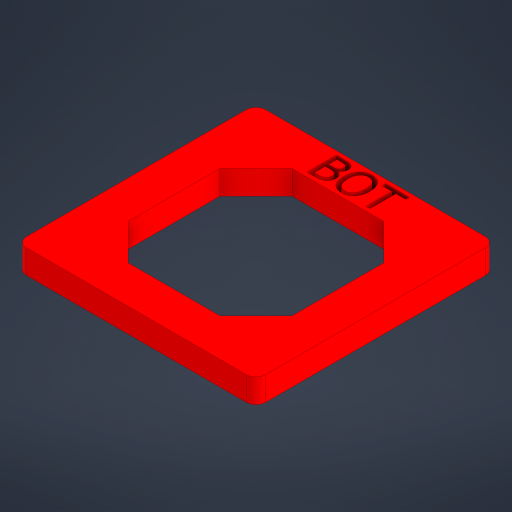
# Autodesk Inventor part: Cube 1x1 V5 Bot Press
Saved by Autodesk Inventor 2023.4 (Build 274418000, 418)
## iProperties
Created: 2022-07-25
Part Number: Cube 1x1 V5 Bot Press
Material: Generic
Document SubType Name: Modeling
Designer: xSibe
Density: 1 g/cm^3
Appearance: Plastic Red
Author: xSibe
Autodesk Inventor part; units mm, degrees
ref_plane "YZ Plane" through (0, 0, 0) normal (1, 0, 0) x (0, 1, 0)
ref_plane "XZ Plane" through (0, 0, 0) normal (0, 1, 0) x (-1, 0, 0)
ref_plane "XY Plane" through (0, 0, 0) normal (0, 0, 1) x (1, 0, 0)
sketch "Sketch1" plane through (0, 0, 0) normal (0, 1, 0) x (-1, 0, 0)
  line L0 (24.9, 24.9) -> (-24.9, 24.9)
  line L1 (-24.9, 24.9) -> (-24.9, -24.9)
  line L2 (-24.9, -24.9) -> (24.9, -24.9)
  line L3 (24.9, -24.9) -> (24.9, 24.9)
  line L4 (24.9, 24.9) -> (-24.9, -24.9) construction
  line L5 (-24.9, 24.9) -> (24.9, -24.9) construction
  line L6 (17.05, 17.05) -> (-17.05, 17.05)
  line L7 (-17.05, 17.05) -> (-17.05, -17.05)
  line L8 (-17.05, -17.05) -> (17.05, -17.05)
  line L9 (17.05, -17.05) -> (17.05, 17.05)
  line L10 (24.9, -24.9) -> (21.9, -24.9)
  line L11 (21.9, -24.9) -> (21.9, -21.9)
  line L12 (21.9, -21.9) -> (24.9, -21.9)
  line L13 (24.9, -21.9) -> (24.9, -24.9)
  circle A0 centre (21.9, -21.9) radius 1.875
  circle A1 centre (21.9, -21.9) radius 2.1063
  circle A2 centre (21.9, -21.9) radius 2.7813
  line L14 (24.9, -24.9) -> (14.4, -24.9)
  line L15 (14.4, -24.9) -> (14.4, -14.4)
  line L16 (14.4, -14.4) -> (24.9, -14.4)
  line L17 (24.9, -14.4) -> (24.9, -24.9)
  line L18 (24.9, -14.4) -> (20.8, -14.4)
  circle A3 centre (20.8, -14.4) radius 2.0725
  circle A4 centre (14.4, -20.8) radius 2.0725
  line L19 (24.9, -24.9) -> (17.05, -24.9)
  line L20 (17.05, -24.9) -> (17.05, -22.55)
  line L21 (22.55, -17.05) -> (24.9, -17.05)
  line L22 (24.9, -17.05) -> (24.9, -24.9)
  line L23 (22.55, -17.05) -> (17.05, -22.55)
  circle A5 centre (21.9, 21.9) radius 2.7813
  circle A6 centre (21.9, 21.9) radius 2.1063
  circle A7 centre (21.9, 21.9) radius 1.875
  circle A8 centre (14.4, 20.8) radius 2.0725
  circle A9 centre (20.8, 14.4) radius 2.0725
  line L24 (17.05, 22.55) -> (22.55, 17.05)
  line L25 (24.9, 17.05) -> (22.55, 17.05)
  line L26 (17.05, 22.55) -> (17.05, 24.9)
  circle A10 centre (-21.9, 21.9) radius 2.7813
  circle A11 centre (-21.9, 21.9) radius 2.1063
  circle A12 centre (-21.9, 21.9) radius 1.875
  circle A13 centre (-20.8, 14.4) radius 2.0725
  circle A14 centre (-14.4, 20.8) radius 2.0725
  line L27 (-22.55, 17.05) -> (-17.05, 22.55)
  line L28 (-17.05, 24.9) -> (-17.05, 22.55)
  line L29 (-22.55, 17.05) -> (-24.9, 17.05)
  circle A15 centre (-21.9, -21.9) radius 2.7813
  circle A16 centre (-21.9, -21.9) radius 2.1063
  circle A17 centre (-21.9, -21.9) radius 1.875
  circle A18 centre (-14.4, -20.8) radius 2.0725
  circle A19 centre (-20.8, -14.4) radius 2.0725
  line L30 (-17.05, -22.55) -> (-22.55, -17.05)
  line L31 (-24.9, -17.05) -> (-22.55, -17.05)
  line L32 (-17.05, -22.55) -> (-17.05, -24.9)
  line L33 (17.05, -22.55) -> (-17.05, -22.55)
  line L34 (-22.55, -17.05) -> (-22.55, 17.05)
  line L35 (-17.05, 22.55) -> (17.05, 22.55)
  line L36 (22.55, 17.05) -> (22.55, -17.05)
  point P0 (0, 0)
  point P1 (-15.5103, -22.55)
  point P2 (14.4, -22.8725)
  point P3 (13.2897, -22.55)
  point P4 (-13.2897, -22.55)
  point P5 (-22.55, -15.5103)
  point P6 (-22.55, -13.2897)
  point P7 (-22.55, 13.2897)
  point P8 (-22.55, 15.5103)
  point P9 (-15.5103, 22.55)
  point P10 (-13.2897, 22.55)
  point P11 (13.2897, 22.55)
  point P12 (15.5103, 22.55)
  point P13 (22.55, -15.5103)
  point P14 (22.55, 15.5103)
  point P15 (22.55, 13.2897)
  point P16 (22.55, -13.2897)
  point P17 (15.5103, -22.55)
  dimension "d0" = 49.8
  dimension "d1" = 49.8
  dimension "d2" = 7.85
  dimension "d3" = 3
  dimension "d4" = 3
  dimension "d5" = 3.75
  dimension "d6" = 4.2125
  dimension "d7" = 0.675
  dimension "d8" = 10.5
  dimension "d9" = 10.5
  dimension "d10" = 4.1
  dimension "d11" = 4.145
  dimension "d12" = 7.85
  dimension "d13" = 7.85
  dimension "d14" = 5.5
  dimension "d15" = 5.5
  dimension "d18" = 360
  constraints: 74 end point, 20 centre point, 10 parallel, 7 perpendicular, 6 coincident, 4 horizontal, 3 point on line, 2 midpoint, 1 symmetric about line, 69 other
  measures "d0" distance of L2.end L1.end
  measures "d1" distance of L1.end L0.end
  measures "d2" distance between parallel lines of L3 L9
  measures "d3" distance of L11.end L12.end
  measures "d4" distance of L10.end L11.end
  measures "d5" diameter of A0
  measures "d6" diameter of A1
  measures "d7" radial gap between concentric circles of A1 A2
  measures "d8" distance of L15.end L16.end
  measures "d9" distance of L14.end L15.end
  measures "d10" distance of L16.end L18.end
  measures "d11" diameter of A3
  measures "d12" distance of point (17.05, -17.05) L21.end
  measures "d13" distance of L19.end point (17.05, -17.05)
  measures "d14" distance of L21.start point (17.05, -17.05)
  measures "d15" distance of L20.end point (17.05, -17.05)
extrude "Extrusion1" add sketch "Sketch1" along normal blind 7.7 contours L3 L25 L24 L26 L0 | L26 L35 A8 A14 L28 L0 | L3 L16 A3 L36 A9 L25 | L28 L27 L29 L1 L0 | L3 L21 L36 A3 L16 | L3 L12 A2 L11 L2 L20 L23 L21 | L29 L34 A13 A19 L31 L1 | L3 L2 L11 A2 L12 | L31 L30 L32 L2 L1 | A2 L11 A1 L12 | L12 A1 L11 A2 | L20 L2 L15 A4 L33 | A1 L11 A0 L12 | L12 A0 L11 A1 | L32 L33 A18 A4 L15 L2 | A0 L11 L12 | L12 L11 A0 | A5 | A6 | A7 | A10 | A11 | A12 | A15 | A16 | A17
extrude "Extrusion2" add sketch "Sketch1" against normal up to surface (7.7 mm away) from surface at 7.7 contours L26 L35 A8 A14 L28 L0 | L3 L16 A3 L36 A9 L25 | L24 L36 A9 A3 L16 L9 L6 L7 L8 L15 A4 L33 A18 L30 L34 A19 A13 L27 L35 A14 A8 | L3 L21 L36 A3 L16 | A3 L36 L16 | L16 L36 A3 | L36 A9 | A9 L36 | L29 L34 A13 A19 L31 L1 | L23 L33 A4 L15 L8 L9 L16 A3 L36 | L36 A3 L16 | L16 A3 L36 | L34 A13 | A13 L34 | L20 L2 L15 A4 L33 | L32 L33 A18 A4 L15 L2 | L34 A19 | A19 L34
chamfer "Chamfer1" [suppressed]
fillet "Fillet1" radius 2 4 edges at (24.9, 3.85, 24.9) (24.9, 3.85, -24.9) (-24.9, 3.85, -24.9) (-24.9, 3.85, 24.9)
chamfer "Chamfer2" distance 0.025 angle 45 8 edges at (0, 7.7, 24.9) (24.3142, 7.7, 24.3142) (24.9, 7.7, 0) (24.3142, 7.7, -24.3142) (0, 7.7, -24.9) (-24.3142, 7.7, -24.3142) (-24.9, 7.7, 0) (-24.3142, 7.7, 24.3142)
extrude "Extrusion3" cut sketch "Sketch1" along normal blind 3 contours A1 L11 A0 L12 | L12 A0 L11 A1 | A0 L11 L12 | L12 L11 A0 | A6 | A7 | A11 | A12 | A16 | A17
extrude "Extrusion4" cut sketch "Sketch1" along normal up to surface (4.7 mm away) from surface at 3 contours A0 L11 L12 | L12 L11 A0 | A7 | A12 | A17
sketch "Sketch2" plane through (0, 7.7, 24.9) normal (0, 0, 1) x (1, 0, 0)
  line L0 (-8.2534, -7.5059) -> (8.2534, -7.5059) construction
  line L1 (8.2534, -7.5059) -> (8.2534, -0.2191) construction
  line L2 (8.2534, -0.2191) -> (-8.2534, -0.2191) construction
  line L3 (-8.2534, -0.2191) -> (-8.2534, -7.5059) construction
  line L4 (-22.9, -3.8625) -> (22.9, -3.8625)
  line L5 (-8.2534, -3.8625) -> (8.2534, -3.8625)
  line L6 (-22.9, -0.025) -> (22.9, -0.025) projected
  line L7 (-22.9, -7.7) -> (-22.9, -0.025) projected
  line L8 (-22.9, -7.7) -> (22.9, -7.7) projected
  line L9 (22.9, -0.025) -> (22.9, -7.7) projected
  point P0 (0, -7.7)
  point P1 (0, -3.8625)
  constraints: 6 midpoint, 4 end point, 1 horizontal, 2 other
extrude "Extrusion5" [suppressed]
pattern_circular "Circular Pattern1" [suppressed]
sketch "Sketch3" plane through (0, 7.7, 0) normal (0, 1, 0) x (1, 0, 0)
  circle A0 centre (21.9, 21.9) radius 1.875 projected
  circle A1 centre (-21.9, -21.9) radius 1.875 projected
  circle A2 centre (-21.9, 21.9) radius 1.875 projected
  circle A3 centre (21.9, -21.9) radius 1.875 projected
  circle A4 centre (-14.4, -20.8) radius 2.0725 projected
  circle A5 centre (14.4, 20.8) radius 2.0725 projected
  circle A6 centre (-14.4, 20.8) radius 2.0725 projected
  line L0 (17.05, -17.05) -> (17.05, 17.05) projected
  line L1 (-17.05, -17.05) -> (17.05, -17.05) projected
  line L2 (-17.05, 17.05) -> (-17.05, -17.05) projected
  line L3 (17.05, 17.05) -> (-17.05, 17.05) projected
  circle A7 centre (14.4, -20.8) radius 2.0725 projected
  line L4 (22.9, -24.875) -> (-22.9, -24.875) projected
  arc A8 (22.9, -24.875) -> (24.875, -22.9) centre (22.9, -22.9) ccw projected
  line L5 (24.875, 22.9) -> (24.875, -22.9) projected
  arc A9 (24.875, 22.9) -> (22.9, 24.875) centre (22.9, 22.9) ccw projected
  line L6 (-22.9, 24.875) -> (22.9, 24.875) projected
  arc A10 (-22.9, 24.875) -> (-24.875, 22.9) centre (-22.9, 22.9) ccw projected
  line L7 (-24.875, -22.9) -> (-24.875, 22.9) projected
  arc A11 (-24.875, -22.9) -> (-22.9, -24.875) centre (-22.9, -22.9) ccw projected
  point P0 (0, 0)
extrude "Extrusion6" add sketch "Sketch3" against normal up to surface (7.7 mm away) contours A0 | A1 | A2 | A3 | L4 A11 L7 A10 L6 A9 L5 A8
sketch "Sketch4" plane through (0, 7.7, 0) normal (0, 1, 0) x (1, 0, 0)
  circle A0 centre (14.4, 20.8) radius 2.0725 projected
  circle A1 centre (-14.4, 20.8) radius 2.0725 projected
  circle A2 centre (-14.4, -20.8) radius 2.0725 projected
  circle A3 centre (14.4, -20.8) radius 2.0725 projected
  line L0 (22.9, -24.875) -> (-22.9, -24.875) projected
  arc A4 (22.9, -24.875) -> (24.875, -22.9) centre (22.9, -22.9) ccw projected
  line L1 (24.875, 22.9) -> (24.875, -22.9) projected
  arc A5 (24.875, 22.9) -> (22.9, 24.875) centre (22.9, 22.9) ccw projected
  line L2 (-22.9, 24.875) -> (22.9, 24.875) projected
  arc A6 (-22.9, 24.875) -> (-24.875, 22.9) centre (-22.9, 22.9) ccw projected
  line L3 (-24.875, -22.9) -> (-24.875, 22.9) projected
  arc A7 (-24.875, -22.9) -> (-22.9, -24.875) centre (-22.9, -22.9) ccw projected
  point P0 (0, 0)
extrude "Extrusion7" add sketch "Sketch4" against normal blind 5.7 contours A0 | A1 | A2 | A3
chamfer "Chamfer3" distance 7.5 angle 45 4 edges at (-17.05, 3.85, 17.05) (17.05, 3.85, 17.05) (17.05, 3.85, -17.05) (-17.05, 3.85, -17.05)
sketch "Sketch5" plane through (0, 7.7, 0) normal (0, 1, 0) x (1, 0, 0)
  line L0 (-9.55, -17.05) -> (9.55, -17.05) projected
  line L1 (-17.05, -9.55) -> (-9.55, -17.05) projected
  line L2 (-17.05, 9.55) -> (-17.05, -9.55) projected
  line L3 (-9.55, 17.05) -> (-17.05, 9.55) projected
  line L4 (9.55, 17.05) -> (-9.55, 17.05) projected
  line L5 (17.05, 9.55) -> (9.55, 17.05) projected
  line L6 (17.05, -9.55) -> (17.05, 9.55) projected
  line L7 (9.55, -17.05) -> (17.05, -9.55) projected
  line L8 (22.9, -24.875) -> (-22.9, -24.875) projected
  arc A0 (22.9, -24.875) -> (24.875, -22.9) centre (22.9, -22.9) ccw projected
  line L9 (24.875, 22.9) -> (24.875, -22.9) projected
  arc A1 (24.875, 22.9) -> (22.9, 24.875) centre (22.9, 22.9) ccw projected
  line L10 (-22.9, 24.875) -> (22.9, 24.875) projected
  arc A2 (-22.9, 24.875) -> (-24.875, 22.9) centre (-22.9, 22.9) ccw projected
  line L11 (-24.875, -22.9) -> (-24.875, 22.9) projected
  arc A3 (-24.875, -22.9) -> (-22.9, -24.875) centre (-22.9, -22.9) ccw projected
  line L12 (22.9, 24.9) -> (-22.9, 24.9) projected
  arc A4 (-22.9, 24.875) -> (-24.875, 22.9) centre (-22.9, 22.9) ccw projected
  arc A5 (-22.9, 24.9) -> (-24.9, 22.9) centre (-22.9, 22.9) ccw projected
  line L13 (-24.9, 22.9) -> (-24.9, -22.9) projected
  arc A6 (-24.9, -22.9) -> (-22.9, -24.9) centre (-22.9, -22.9) ccw projected
  arc A7 (-24.9, -22.9) -> (-22.9, -24.9) centre (-22.9, -22.9) ccw projected
  line L14 (-22.9, -24.9) -> (22.9, -24.9) projected
  line L15 (-22.9, -24.9) -> (22.9, -24.9) projected
  arc A8 (22.9, -24.9) -> (24.9, -22.9) centre (22.9, -22.9) ccw projected
  arc A9 (22.9, -24.9) -> (24.9, -22.9) centre (22.9, -22.9) ccw projected
  line L16 (24.9, -22.9) -> (24.9, 22.9) projected
  line L17 (24.9, -22.9) -> (24.9, 22.9) projected
  arc A10 (24.9, 22.9) -> (22.9, 24.9) centre (22.9, 22.9) ccw projected
  arc A11 (24.9, 22.9) -> (22.9, 24.9) centre (22.9, 22.9) ccw projected
  line L18 (0, 17.05) -> (0, 24.9)
  line L19 (-10, 17.05) -> (10, 17.05)
  line L20 (10, 17.05) -> (10, 24.9)
  line L21 (10, 24.9) -> (-10, 24.9)
  line L22 (-10, 24.9) -> (-10, 17.05)
  line L23 (-10, 17.05) -> (10, 24.9) construction
  line L24 (10, 17.05) -> (-10, 24.9) construction
  line L25 (-10, 24.9) -> (10, 24.9) construction
  line L26 (10, 24.9) -> (10, 17.05) construction
  line L27 (10, 17.05) -> (-10, 17.05) construction
  line L28 (-10, 17.05) -> (-10, 24.9) construction
  spline S0 degree 2 poles (-3.1365, 19.7985) (-3.1365, 19.3437) (-3.4825, 18.6467) (-3.7692, 18.4193) knots 0 0 0 1 2 2 2
  spline S1 degree 2 poles (-3.7692, 18.4193) (-4.1153, 18.1524) (-4.9013, 17.925) (-5.5241, 17.925) knots 0 0 0 1 2 2 2
  line L29 (-5.5241, 17.925) -> (-7.274, 17.925)
  line L30 (-7.274, 17.925) -> (-7.274, 24.025)
  line L31 (-7.274, 24.025) -> (-5.6576, 24.025)
  spline S2 degree 2 poles (-5.6576, 24.025) (-5.0051, 24.025) (-4.3526, 23.941) (-4.056, 23.7778) knots 0 0 0 1 2 2 2
  spline S3 degree 2 poles (-4.056, 23.7778) (-3.7248, 23.6048) (-3.4232, 23.0363) (-3.4232, 22.6508) knots 0 0 0 1 2 2 2
  spline S4 degree 2 poles (-3.4232, 22.6508) (-3.4232, 22.2207) (-3.878, 21.5385) (-4.2784, 21.3457) knots 0 0 0 1 2 2 2
  line L32 (-4.2784, 21.3457) -> (-4.2784, 21.3161)
  spline S5 degree 2 poles (-4.2784, 21.3161) (-3.7346, 21.1678) (-3.1365, 20.3818) (-3.1365, 19.7985) knots 0 0 0 1 2 2 2
  spline S6 degree 2 poles (-3.9818, 19.7639) (-3.9818, 20.1099) (-4.1795, 20.5548) (-4.4761, 20.713) knots 0 0 0 1 2 2 2
  spline S7 degree 2 poles (-4.4761, 20.713) (-4.6689, 20.8119) (-5.1237, 20.8712) (-5.5439, 20.8712) knots 0 0 0 1 2 2 2
  line L33 (-5.5439, 20.8712) -> (-6.4633, 20.8712)
  line L34 (-6.4633, 20.8712) -> (-6.4633, 18.6171)
  line L35 (-6.4633, 18.6171) -> (-5.8059, 18.6171)
  spline S8 degree 2 poles (-5.8059, 18.6171) (-5.272, 18.6171) (-4.659, 18.7159) (-4.4218, 18.8741) knots 0 0 0 1 2 2 2
  spline S9 degree 2 poles (-4.4218, 18.8741) (-4.1944, 19.0372) (-3.9818, 19.4426) (-3.9818, 19.7639) knots 0 0 0 1 2 2 2
  spline S10 degree 2 poles (-4.2685, 22.5371) (-4.2685, 22.7546) (-4.4168, 23.0808) (-4.5799, 23.1748) knots 0 0 0 1 2 2 2
  spline S11 degree 2 poles (-4.5799, 23.1748) (-4.7777, 23.2835) (-5.2572, 23.3329) (-5.6872, 23.3329) knots 0 0 0 1 2 2 2
  line L36 (-5.6872, 23.3329) -> (-6.4633, 23.3329)
  line L37 (-6.4633, 23.3329) -> (-6.4633, 21.5484)
  line L38 (-6.4633, 21.5484) -> (-5.5439, 21.5484)
  spline S12 degree 2 poles (-5.5439, 21.5484) (-5.1632, 21.5484) (-4.8024, 21.6275) (-4.6096, 21.7511) knots 0 0 0 1 2 2 2
  spline S13 degree 2 poles (-4.6096, 21.7511) (-4.4218, 21.8697) (-4.2685, 22.2504) (-4.2685, 22.5371) knots 0 0 0 1 2 2 2
  spline S14 degree 2 poles (1.9847, 23.328) (2.3308, 22.9227) (2.7163, 21.7363) (2.7163, 20.975) knots 0 0 0 1 2 2 2
  spline S15 degree 2 poles (2.7163, 20.975) (2.7163, 20.2335) (2.3406, 19.0323) (1.9847, 18.6269) knots 0 0 0 1 2 2 2
  spline S16 degree 2 poles (1.9847, 18.6269) (1.609, 18.2018) (0.6154, 17.7965) (0.0173, 17.7965) knots 0 0 0 1 2 2 2
  spline S17 degree 2 poles (0.0173, 17.7965) (-0.6006, 17.7965) (-1.5893, 18.2167) (-1.9501, 18.6269) knots 0 0 0 1 2 2 2
  spline S18 degree 2 poles (-1.9501, 18.6269) (-2.3011, 19.0323) (-2.6768, 20.2236) (-2.6768, 20.975) knots 0 0 0 1 2 2 2
  spline S19 degree 2 poles (-2.6768, 20.975) (-2.6768, 21.7412) (-2.2962, 22.9078) (-1.9452, 23.328) knots 0 0 0 1 2 2 2
  spline S20 degree 2 poles (-1.9452, 23.328) (-1.5893, 23.7333) (-0.5957, 24.1535) (0.0173, 24.1535) knots 0 0 0 1 2 2 2
  spline S21 degree 2 poles (0.0173, 24.1535) (0.6402, 24.1535) (1.6387, 23.7185) (1.9847, 23.328) knots 0 0 0 1 2 2 2
  spline S22 degree 2 poles (1.871, 20.975) (1.871, 21.5781) (1.609, 22.5124) (1.3718, 22.8188) knots 0 0 0 1 2 2 2
  spline S23 degree 2 poles (1.3718, 22.8188) (1.1295, 23.1352) (0.4474, 23.4516) (0.0222, 23.4516) knots 0 0 0 1 2 2 2
  spline S24 degree 2 poles (0.0222, 23.4516) (-0.4177, 23.4516) (-1.0801, 23.1451) (-1.3322, 22.8188) knots 0 0 0 1 2 2 2
  spline S25 degree 2 poles (-1.3322, 22.8188) (-1.5744, 22.5074) (-1.8315, 21.5682) (-1.8315, 20.975) knots 0 0 0 1 2 2 2
  spline S26 degree 2 poles (-1.8315, 20.975) (-1.8315, 19.7738) (-0.8231, 18.4984) (0.0222, 18.4984) knots 0 0 0 1 2 2 2
  spline S27 degree 2 poles (0.0222, 18.4984) (0.8675, 18.4984) (1.871, 19.7738) (1.871, 20.975) knots 0 0 0 1 2 2 2
  line L39 (5.0298, 17.925) -> (5.0298, 23.3033)
  line L40 (5.0298, 23.3033) -> (2.9833, 23.3033)
  line L41 (2.9833, 23.3033) -> (2.9833, 24.025)
  line L42 (2.9833, 24.025) -> (7.887, 24.025)
  line L43 (7.887, 24.025) -> (7.887, 23.3033)
  line L44 (7.887, 23.3033) -> (5.8405, 23.3033)
  line L45 (5.8405, 23.3033) -> (5.8405, 17.925)
  line L46 (5.8405, 17.925) -> (5.0298, 17.925)
  point P0 (0, 0)
  point P1 (0, 20.975)
  point P2 (-10, 24.875)
  point P3 (10, 24.875)
  dimension "d49" = 20
  constraints: 14 end point, 5 midpoint, 2 coincident, 2 parallel, 1 horizontal, 1 perpendicular, 1 point on line, 2 other
  measures "d49" distance of L21.end L20.end
extrude "Extrusion8" cut sketch "Sketch5" against normal blind 2.7 contours L0 L7 L6 L5 L19 L20 L10 A1 L9 A0 L8 A3 L11 A2 L22 L3 L2 L1 | L19 L22 L10 L18 S20 S19 S18 S17 L4 | L4 L18 S17 S16 S15 S14 S21 S20 L10 L20 L19 | S17 S18 S19 S20 L18 S24 S25 S26 | L18 S26 S27 S22 S23 S24 S20 S21 S14 S15 S16 S17 | L22 L12 L18 L10 | L10 A2 L11 A3 L8 A0 L9 A1 L20 L12 A10 L16 A8 L14 A6 L13 A5 L22 | L10 L18 L12 L20 | S26 S25 S24 L18 | L18 S24 S23 S22 S27 S26 | S0 S1 L29 L30 L31 S2 S3 S4 L32 S5 | S9 S8 L35 L34 L33 S7 S6 | S13 S12 L38 L37 L36 S11 S10 | L39 L40 L41 L42 L43 L44 L45 L46
extrude "Extrusion9" cut sketch "Sketch5" against normal blind 2.5 from surface at -2.7 contours S17 S18 S19 S20 L18 S24 S25 S26 | L18 S26 S27 S22 S23 S24 S20 S21 S14 S15 S16 S17 | S0 S1 L29 L30 L31 S2 S3 S4 L32 S5 | L39 L40 L41 L42 L43 L44 L45 L46
equation "\"d15\" = d14"
body "Solid1"
